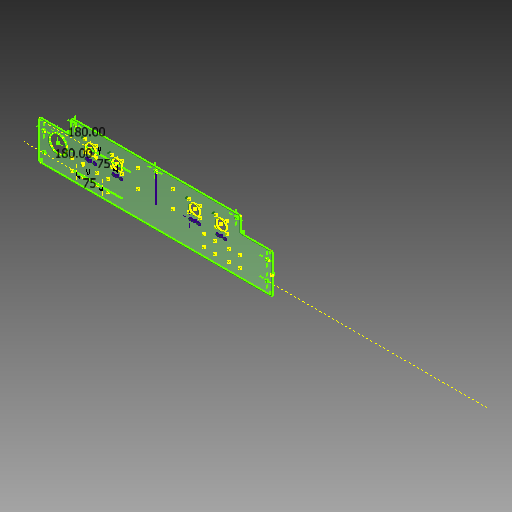
# Autodesk Inventor part: Rear Extruder Panel
Saved by Autodesk Inventor 2018 (Build 220112000, 112)
## iProperties
Created: 2016-06-26
Part Number: Rear Extruder Panel
Material: Polycarbonate, Smoke
Document SubType Name: Modeling
Designer: joshmamo
Density: 1.2 g/cm^3
Appearance: Polycarbonate - Clear(1)
Author: joshmamo
Autodesk Inventor part; units mm, degrees
ref_plane "YZ Plane" through (0, 0, 0) normal (1, 0, 0) x (0, 1, 0)
ref_plane "XZ Plane" through (0, 0, 0) normal (0, 1, 0) x (-1, 0, 0)
ref_plane "XY Plane" through (0, 0, 0) normal (0, 0, 1) x (1, 0, 0)
sketch "Sketch2" plane through (0, 0, 0) normal (0, 0, 1) x (1, 0, 0)
  line L0 (-94.6, 98.6888) -> (-564.8, 98.6888)
  line L1 (-89.6, 60.678) -> (-89.6, 93.6888)
  line L2 (-5, 55.678) -> (-84.6, 55.678)
  line L3 (0, -48.6888) -> (0, 48.6888)
  line L4 (-655, -53.6888) -> (-5, -53.6888)
  line L5 (-660, 50.6888) -> (-660, -48.6888)
  line L6 (-574.8, 55.6888) -> (-655, 55.6888)
  line L7 (-569.8, 93.6888) -> (-569.8, 60.6888)
  line L8 (-94.6, 98.6888) -> (-564.8, 98.6888)
  line L9 (-569.8, 93.6888) -> (-569.8, 60.6888)
  line L10 (-574.8, 55.6888) -> (-655, 55.6888)
  line L11 (-660, 50.6888) -> (-660, -48.6888)
  line L12 (-655, -53.6888) -> (-5, -53.6888)
  line L13 (0, -48.6888) -> (0, 50.678)
  line L14 (-5, 55.678) -> (-84.6, 55.678)
  line L15 (-89.6, 60.678) -> (-89.6, 93.6888)
  arc A0 (-89.6, 93.6888) -> (-94.6, 98.6888) centre (-94.6, 93.6888) ccw
  arc A1 (-89.6, 60.678) -> (-84.6, 55.678) centre (-84.6, 60.678) ccw
  arc A2 (0, 50.678) -> (-5, 55.678) centre (-5, 50.678) ccw
  arc A3 (-5, -53.6888) -> (0, -48.6888) centre (-5, -48.6888) ccw
  arc A4 (-660, -48.6888) -> (-655, -53.6888) centre (-655, -48.6888) ccw
  arc A5 (-655, 55.6888) -> (-660, 50.6888) centre (-655, 50.6888) ccw
  arc A6 (-574.8, 55.6888) -> (-569.8, 60.6888) centre (-574.8, 60.6888) ccw
  arc A7 (-564.8, 98.6888) -> (-569.8, 93.6888) centre (-564.8, 93.6888) ccw
  circle A8 centre (-605.9899, 16.8231) radius 24.5048
  line L16 (-17.508, -23.922) -> (609.984, -23.922) construction
  circle A9 centre (-645, 28.378) radius 2.55
  circle A10 centre (-645, -23.922) radius 2.55
  circle A11 centre (-557.8, 87.2888) radius 2.55
  circle A12 centre (-329.8, 87.2888) radius 2.55
  circle A13 centre (-101.8, 87.2888) radius 2.55
  circle A14 centre (-15, 28.378) radius 2.55
  circle A15 centre (-15, -23.922) radius 2.55
  point P0 (0, 0)
  point P1 (-581.4851, 16.8231)
  point P2 (-605.9899, 41.3279)
  point P3 (-560.308, 87.2888)
  point P4 (-557.8, 89.7968)
  point P5 (-645, 30.8968)
  point P6 (-647.508, 28.3888)
  point P7 (-329.8, 89.7968)
  point P8 (-332.308, 87.2888)
  point P9 (-101.8, 89.7968)
  point P10 (-104.308, 87.2888)
  point P11 (-15, 30.886)
  point P12 (-17.508, 28.378)
  point P13 (-15, -21.414)
  constraints: 37 end point, 16 point on circle, 15 centre point, 14 point on line, 1 horizontal, 1 vertical alignment, 2 other
sketch "Sketch3" plane through (0, 0, 0) normal (0, 0, 1) x (1, 0, 0)
  line L0 (-94.6, 98.6888) -> (-564.8, 98.6888)
  arc A0 (-564.8, 98.6888) -> (-569.8, 93.6888) centre (-564.8, 93.6888) ccw
  line L1 (-94.6, 98.6888) -> (-564.8, 98.6888)
  line L2 (-569.8, 93.6888) -> (-569.8, 60.6888)
  arc A1 (-574.8, 55.6888) -> (-569.8, 60.6888) centre (-574.8, 60.6888) ccw
  line L3 (-574.8, 55.6888) -> (-655, 55.6888)
  arc A2 (-655, 55.6888) -> (-660, 50.6888) centre (-655, 50.6888) ccw
  line L4 (-660, 50.6888) -> (-660, -48.6888)
  arc A3 (-660, -48.6888) -> (-655, -53.6888) centre (-655, -48.6888) ccw
  line L5 (-655, -53.6888) -> (-5, -53.6888)
  circle A4 centre (-605.9899, 16.8231) radius 24.5048
  circle A5 centre (-645, -23.922) radius 2.55
  circle A6 centre (-645, 28.378) radius 2.55
  circle A7 centre (-557.8, 87.2888) radius 2.55
  circle A8 centre (-329.8, 87.2888) radius 2.55
  circle A9 centre (-101.8, 87.2888) radius 2.55
  circle A10 centre (-15, 28.378) radius 2.55
  circle A11 centre (-15, -23.922) radius 2.55
  arc A12 (-5, -53.6888) -> (0, -48.6888) centre (-5, -48.6888) ccw
  line L6 (0, -48.6888) -> (0, 48.6888)
  arc A13 (0, 50.678) -> (-5, 55.678) centre (-5, 50.678) ccw
  line L7 (-5, 55.678) -> (-84.6, 55.678)
  arc A14 (-89.6, 60.678) -> (-84.6, 55.678) centre (-84.6, 60.678) ccw
  line L8 (-89.6, 60.678) -> (-89.6, 93.6888)
  arc A15 (-89.6, 93.6888) -> (-94.6, 98.6888) centre (-94.6, 93.6888) ccw
  point P0 (0, 0)
  constraints: 18 end point, 16 centre point, 16 point on circle
sketch "Sketch4" plane through (0, 0, 0) normal (0, 0, 1) x (1, 0, 0)
  line L0 (-94.6, 98.6888) -> (-564.8, 98.6888) projected
  arc A0 (-89.6, 93.6888) -> (-94.6, 98.6888) centre (-94.6, 93.6888) ccw projected
  line L1 (-89.6, 60.678) -> (-89.6, 93.6888) projected
  arc A1 (-89.6, 60.678) -> (-84.6, 55.678) centre (-84.6, 60.678) ccw projected
  line L2 (-5, 55.678) -> (-84.6, 55.678) projected
  arc A2 (0, 50.678) -> (-5, 55.678) centre (-5, 50.678) ccw projected
  line L3 (0, -48.6888) -> (0, 50.678) projected
  arc A3 (-5, -53.6888) -> (0, -48.6888) centre (-5, -48.6888) ccw projected
  line L4 (-655, -53.6888) -> (-5, -53.6888) projected
  arc A4 (-660, -48.6888) -> (-655, -53.6888) centre (-655, -48.6888) ccw projected
  line L5 (-660, 50.6888) -> (-660, -48.6888) projected
  arc A5 (-655, 55.6888) -> (-660, 50.6888) centre (-655, 50.6888) ccw projected
  line L6 (-574.8, 55.6888) -> (-655, 55.6888) projected
  arc A6 (-574.8, 55.6888) -> (-569.8, 60.6888) centre (-574.8, 60.6888) ccw projected
  line L7 (-569.8, 93.6888) -> (-569.8, 60.6888) projected
  arc A7 (-564.8, 98.6888) -> (-569.8, 93.6888) centre (-564.8, 93.6888) ccw projected
  point P0 (0, 0)
extrude "Extrusion1" add sketch "Sketch4" along normal blind 3
extrude "Extrusion2" cut sketch "Sketch3" along normal blind 3
sketch "Sketch5" plane through (0, 0, 0) normal (0, 0, -1) x (-1, 0, 0)
  line L0 (562.0823, -27.0183) -> (423.5029, -27.0183)
  line L1 (562.0823, -27.0183) -> (700.6617, -27.0183) construction
  line L2 (524.9252, 49.2029) -> (403.8589, 49.2029)
  line L3 (524.9252, 49.2029) -> (645.9914, 49.2029) construction
  line L4 (403.8589, 49.2029) -> (514.2755, 49.2029)
  line L5 (514.2755, 49.2029) -> (439.2755, 49.2029)
  line L6 (554.3408, -27.0183) -> (479.3408, -27.0183)
  point P0 (0, 0)
  dimension "d13" = 180
  dimension "d14" = 180
  dimension "d15" = 75
  dimension "d16" = 75
  constraints: 14 end point, 4 point on line, 2 collinear, 2 horizontal
  measures "d13" angle of L0 L1
  measures "d14" angle of L2 L3
  measures "d15" distance of L4.end L5.end
  measures "d16" distance of L6.start L6.end
sketch "Sketch6" plane through (0, 0, 0) normal (0, 0, -1) x (-1, 0, 0)
  circle A0 centre (529.7755, 64.7029) radius 1.7254
  circle A1 centre (498.7755, 64.7029) radius 1.6
  circle A2 centre (454.7755, 64.7029) radius 1.7254
  circle A3 centre (423.7755, 64.7029) radius 1.6
  spline S0 degree 3 number of poles 70
  circle A4 centre (498.7755, 33.6984) radius 1.6
  circle A5 centre (529.7755, 33.6984) radius 1.6
  circle A6 centre (529.7755, 64.7029) radius 1.6
  circle A7 centre (498.7755, 64.7029) radius 1.6
  circle A8 centre (454.7755, 33.6984) radius 1.6
  circle A9 centre (423.7755, 33.6984) radius 1.6
  circle A10 centre (454.7755, 64.7029) radius 1.6
  circle A11 centre (423.7755, 64.7029) radius 1.6
  circle A12 centre (329.8, 87.2888) radius 2.55
  line L0 (329.8, 87.2888) -> (329.8, 46.3988)
  point P0 (0, 0)
  point P1 (569.8408, -11.5183)
  point P2 (538.8408, -11.5183)
  point P3 (494.8408, -11.5183)
  point P4 (463.8408, -11.5183)
  point P5 (569.8408, -42.5229)
  point P6 (538.8408, -42.5229)
  point P7 (494.8408, -42.5229)
  point P8 (463.8408, -42.5229)
  point P9 (497.2709, 33.6984)
  point P10 (129.8245, 64.7029)
  point P11 (204.8245, 64.7029)
  point P12 (235.8245, 64.7029)
  point P13 (160.8245, 33.6984)
  point P14 (129.8245, 33.6984)
  point P15 (160.8245, 64.7029)
  point P16 (204.8245, 33.6984)
  point P17 (235.8245, 33.6984)
  dimension "d25" = 3.2
  dimension "d26" = 3.2
  dimension "d27" = 3.2
  dimension "d28" = 3.2
  dimension "d29" = 3.2
  dimension "d30" = 3.2
  dimension "d31" = 3.2
  dimension "d32" = 3.2
  constraints: 8 centre point, 8 symmetric about line, 4 coincident, 2 end point, 1 vertical
  measures "d25" diameter of A4
  measures "d26" diameter of A5
  measures "d27" diameter of A6
  measures "d28" diameter of A7
  measures "d29" diameter of A8
  measures "d30" diameter of A9
  measures "d31" diameter of A10
  measures "d32" diameter of A11
sketch "Sketch7" plane through (0, 0, 0) normal (0, 0, -1) x (-1, 0, 0)
  point P0 (0, 0)
  point P1 (554.3408, -27.0183)
  point P2 (479.3408, -27.0183)
  point P3 (439.2755, 49.2029)
  point P4 (514.2755, 49.2029)
sketch "Sketch8" plane through (0, 0, 0) normal (0, 0, -1) x (-1, 0, 0)
  circle A0 centre (439.2755, 49.2029) radius 14.5 projected
  circle A1 centre (514.2755, 49.2029) radius 14.5 projected
  circle A2 centre (329.8, 87.2888) radius 2.55 projected
  line L0 (329.8, 87.2888) -> (329.8, 25.8956)
  circle A3 centre (220.3245, 49.2029) radius 14.5
  circle A4 centre (145.3245, 49.2029) radius 14.5
  point P0 (0, 0)
  constraints: 2 end point, 2 symmetric about line, 1 vertical, 2 other
extrude "Extrusion3" cut sketch "Sketch8" against normal through all contours A0 | A1 | A3 | A4
sketch "Sketch9" plane through (0, 0, 0) normal (0, 0, -1) x (-1, 0, 0)
  circle A0 centre (329.8, 87.2888) radius 2.55 projected
  line L0 (329.8, 87.2888) -> (329.8, 5.9494)
  point P0 (0, 0)
  constraints: 2 end point, 1 vertical
hole "Hole2" at (-423.7755, 64.7029, 0) at (-423.7755, 33.6984, 0) at (-454.7755, 33.6984, 0) at (-454.7755, 64.7029, 0) at (-498.7755, 33.6984, 0) at (-498.7755, 64.7029, 0) at (-529.7755, 64.7029, 0) at (-529.7755, 33.6984, 0) at (-235.8245, 64.7029, 0) at (-204.8245, 64.7029, 0) at (-204.8245, 33.6984, 0) at (-235.8245, 33.6984, 0) at (-160.8245, 33.6984, 0) at (-160.8245, 64.7029, 0) at (-129.8245, 64.7029, 0) at (-129.8245, 33.6984, 0) direction (0, 0, 1) diameter 3 end through all
sketch "Sketch10" plane through (0, 0, 0) normal (0, 0, -1) x (-1, 0, 0)
  line L0 (329.8, 87.2888) -> (329.8, 5.9494) projected
  line L1 (329.8, 68.5151) -> (279.8, 68.5151)
  line L2 (329.8, 68.5151) -> (329.8, 18.5151)
  line L3 (329.8, 18.5151) -> (279.8, 18.5151)
  line L4 (279.8, 18.5151) -> (379.8, 18.5151)
  line L5 (379.8, 18.5151) -> (379.8, 68.5151)
  line L6 (329.8, 0) -> (91.883, 0)
  line L7 (91.883, 0) -> (91.883, -31.05)
  line L8 (91.883, -31.05) -> (122.933, -31.05)
  line L9 (91.883, 0) -> (122.933, 0)
  line L10 (122.933, 0) -> (162.933, 0)
  line L11 (162.933, 0) -> (162.933, -31.05)
  line L12 (162.933, -31.05) -> (193.983, -31.05)
  line L13 (567.717, 0) -> (567.717, -31.05)
  line L14 (567.717, -31.05) -> (536.667, -31.05)
  line L15 (496.667, 0) -> (496.667, -31.05)
  line L16 (496.667, -31.05) -> (465.617, -31.05)
  point P0 (0, 0)
  point P1 (193.983, 0)
  point P2 (536.667, 0)
  point P3 (465.617, 0)
  dimension "d49" = 50
  dimension "d50" = 50
  dimension "d51" = 100
  dimension "d52" = 31.05
  dimension "d53" = 31.05
  dimension "d54" = 40
  dimension "d55" = 31.05
  dimension "d56" = 31.05
  constraints: 32 end point, 8 symmetric about line, 5 point on line, 4 perpendicular, 3 horizontal
  measures "d49" distance of L1.start L1.end
  measures "d50" distance of L1.start L2.end
  measures "d51" distance of L3.end L4.end
  measures "d52" distance of L6.end L7.end
  measures "d53" distance of L7.end L8.end
  measures "d54" distance of L9.end L10.end
  measures "d55" distance of L11.start L11.end
  measures "d56" distance of L11.end L12.end
hole "Hole3" at (-91.883, 0, 0) at (-91.883, -31.05, 0) at (-122.933, -31.05, 0) at (-122.933, 0, 0) at (-162.933, 0, 0) at (-162.933, -31.05, 0) at (-193.983, -31.05, 0) at (-193.983, 0, 0) at (-279.8, 18.5151, 0) at (-279.8, 68.5151, 0) at (-379.8, 68.5151, 0) at (-379.8, 18.5151, 0) at (-496.667, 0, 0) at (-496.667, -31.05, 0) at (-465.617, -31.05, 0) at (-465.617, 0, 0) at (-536.667, 0, 0) at (-567.717, 0, 0) at (-567.717, -31.05, 0) at (-536.667, -31.05, 0) direction (0, 0, 1) diameter 3 end through all
sketch "Sketch11" plane through (0, 0, 0) normal (0, 0, -1) x (-1, 0, 0)
  circle A0 centre (567.717, -31.05) radius 1.5 projected
  circle A1 centre (536.667, 0) radius 1.5 projected
  circle A2 centre (465.617, -31.05) radius 1.5 projected
  circle A3 centre (496.667, 0) radius 1.5 projected
  circle A4 centre (379.8, 68.5151) radius 1.5 projected
  circle A5 centre (279.8, 18.5151) radius 1.5 projected
  circle A6 centre (193.983, -31.05) radius 1.5 projected
  circle A7 centre (162.933, 0) radius 1.5 projected
  circle A8 centre (122.933, -31.05) radius 1.5 projected
  circle A9 centre (91.883, 0) radius 1.5 projected
  circle A10 centre (91.883, -31.05) radius 1.5 projected
  circle A11 centre (122.933, 0) radius 1.5 projected
  circle A12 centre (162.933, -31.05) radius 1.5 projected
  circle A13 centre (193.983, 0) radius 1.5 projected
  circle A14 centre (279.8, 68.5151) radius 1.5 projected
  circle A15 centre (379.8, 18.5151) radius 1.5 projected
  circle A16 centre (496.667, -31.05) radius 1.5 projected
  circle A17 centre (465.617, 0) radius 1.5 projected
  circle A18 centre (567.717, 0) radius 1.5 projected
  circle A19 centre (536.667, -31.05) radius 1.5 projected
  circle A20 centre (129.8245, 64.7029) radius 1.5 projected
  circle A21 centre (160.8245, 33.6984) radius 1.5 projected
  circle A22 centre (204.8245, 33.6984) radius 1.5 projected
  circle A23 centre (235.8245, 64.7029) radius 1.5 projected
  circle A24 centre (529.7755, 64.7029) radius 1.5 projected
  circle A25 centre (498.7755, 33.6984) radius 1.5 projected
  circle A26 centre (454.7755, 33.6984) radius 1.5 projected
  circle A27 centre (423.7755, 64.7029) radius 1.5 projected
  circle A28 centre (423.7755, 33.6984) radius 1.5 projected
  circle A29 centre (454.7755, 64.7029) radius 1.5 projected
  circle A30 centre (498.7755, 64.7029) radius 1.5 projected
  circle A31 centre (529.7755, 33.6984) radius 1.5 projected
  circle A32 centre (204.8245, 64.7029) radius 1.5 projected
  circle A33 centre (235.8245, 33.6984) radius 1.5 projected
  circle A34 centre (160.8245, 64.7029) radius 1.5 projected
  circle A35 centre (129.8245, 33.6984) radius 1.5 projected
  circle A36 centre (220.3245, 49.2029) radius 14.5 projected
  circle A37 centre (439.2755, 49.2029) radius 14.5 projected
  circle A38 centre (514.2755, 49.2029) radius 14.5 projected
  circle A39 centre (145.3245, 49.2029) radius 14.5 projected
  circle A40 centre (15, -23.922) radius 2.55 projected
  circle A41 centre (101.8, 87.2888) radius 2.55 projected
  circle A42 centre (557.8, 87.2888) radius 2.55 projected
  circle A43 centre (645, -23.922) radius 2.55 projected
  circle A44 centre (645, 28.378) radius 2.55 projected
  circle A45 centre (329.8, 87.2888) radius 2.55 projected
  circle A46 centre (15, 28.378) radius 2.55 projected
  circle A47 centre (605.9899, 16.8231) radius 24.5048 projected
  line L0 (94.6, 98.6888) -> (564.8, 98.6888) projected
  arc A48 (94.6, 98.6888) -> (89.6, 93.6888) centre (94.6, 93.6888) ccw projected
  line L1 (89.6, 60.678) -> (89.6, 93.6888) projected
  arc A49 (84.6, 55.678) -> (89.6, 60.678) centre (84.6, 60.678) ccw projected
  line L2 (5, 55.678) -> (84.6, 55.678) projected
  arc A50 (5, 55.678) -> (0, 50.678) centre (5, 50.678) ccw projected
  line L3 (0, -48.6888) -> (0, 50.678) projected
  arc A51 (0, -48.6888) -> (5, -53.6888) centre (5, -48.6888) ccw projected
  line L4 (655, -53.6888) -> (5, -53.6888) projected
  arc A52 (655, -53.6888) -> (660, -48.6888) centre (655, -48.6888) ccw projected
  line L5 (660, 50.6888) -> (660, -48.6888) projected
  arc A53 (660, 50.6888) -> (655, 55.6888) centre (655, 50.6888) ccw projected
  line L6 (574.8, 55.6888) -> (655, 55.6888) projected
  arc A54 (569.8, 60.6888) -> (574.8, 55.6888) centre (574.8, 60.6888) ccw projected
  line L7 (569.8, 93.6888) -> (569.8, 60.6888) projected
  arc A55 (569.8, 93.6888) -> (564.8, 98.6888) centre (564.8, 93.6888) ccw projected
  circle A56 centre (145.3245, 19.7029) radius 1.6
  line L8 (137.8245, 17.6529) -> (131.6245, 17.6529)
  line L9 (137.8245, 21.7529) -> (137.8245, 17.6529)
  line L10 (131.6245, 21.7529) -> (137.8245, 21.7529)
  line L11 (131.6245, 17.6529) -> (131.6245, 21.7529)
  circle A57 centre (145.3245, 19.7029) radius 1.6
  line L12 (152.8245, 17.6529) -> (159.0245, 17.6529)
  line L13 (159.0245, 17.6529) -> (159.0245, 21.7529)
  line L14 (159.0245, 21.7529) -> (152.8245, 21.7529)
  line L15 (152.8245, 21.7529) -> (152.8245, 17.6529)
  line L16 (212.8245, 17.6529) -> (206.6245, 17.6529)
  line L17 (206.6245, 17.6529) -> (206.6245, 21.7529)
  line L18 (206.6245, 21.7529) -> (212.8245, 21.7529)
  line L19 (212.8245, 21.7529) -> (212.8245, 17.6529)
  circle A58 centre (220.3245, 19.7029) radius 1.6
  line L20 (227.8245, 17.6529) -> (234.0245, 17.6529)
  line L21 (234.0245, 17.6529) -> (234.0245, 21.7529)
  line L22 (234.0245, 21.7529) -> (227.8245, 21.7529)
  line L23 (227.8245, 21.7529) -> (227.8245, 17.6529)
  circle A59 centre (439.2755, 19.7029) radius 1.6
  line L24 (431.7755, 21.7529) -> (431.7755, 17.6529)
  line L25 (431.7755, 17.6529) -> (425.5755, 17.6529)
  line L26 (425.5755, 17.6529) -> (425.5755, 21.7529)
  line L27 (425.5755, 21.7529) -> (431.7755, 21.7529)
  line L28 (446.7755, 21.7529) -> (446.7755, 17.6529)
  line L29 (446.7755, 17.6529) -> (452.9755, 17.6529)
  line L30 (452.9755, 17.6529) -> (452.9755, 21.7529)
  line L31 (452.9755, 21.7529) -> (446.7755, 21.7529)
  line L32 (506.7755, 17.6529) -> (500.5755, 17.6529)
  line L33 (506.7755, 21.7529) -> (506.7755, 17.6529)
  line L34 (500.5755, 21.7529) -> (506.7755, 21.7529)
  line L35 (500.5755, 17.6529) -> (500.5755, 21.7529)
  circle A60 centre (514.2755, 19.7029) radius 1.6
  line L36 (521.7755, 17.6529) -> (527.9755, 17.6529)
  line L37 (527.9755, 17.6529) -> (527.9755, 21.7529)
  line L38 (527.9755, 21.7529) -> (521.7755, 21.7529)
  line L39 (521.7755, 21.7529) -> (521.7755, 17.6529)
  point P0 (0, 0)
  constraints: 64 end point, 16 horizontal, 16 vertical, 5 centre point, 43 other
sketch "Sketch13" plane through (0, 0, 0) normal (0, 0, -1) x (-1, 0, 0)
  circle A0 centre (145.3245, 19.7029) radius 1.6 projected
  line L0 (152.9245, 21.2029) -> (158.9245, 21.2029) projected
  line L1 (158.9245, 21.2029) -> (158.9245, 18.2029) projected
  line L2 (152.9245, 18.2029) -> (152.9245, 21.2029) projected
  line L3 (158.9245, 18.2029) -> (152.9245, 18.2029) projected
  line L4 (137.7245, 21.2029) -> (137.7245, 18.2029) projected
  line L5 (131.7245, 21.2029) -> (137.7245, 21.2029) projected
  line L6 (131.7245, 18.2029) -> (131.7245, 21.2029) projected
  line L7 (137.7245, 18.2029) -> (131.7245, 18.2029) projected
  point P0 (0, 0)
extrude "Extrusion5" cut sketch "Sketch13" against normal through all
pattern_linear "Rectangular Pattern1" count 2 spacing 75 along (-1, 0, 0) of "Extrusion5"
pattern_linear "Rectangular Pattern2" count 2 spacing 294 along (-1, 0, 0) of "Extrusion5"
pattern_linear "Rectangular Pattern3" count 2 spacing 75 along (-1, 0, 0) of "Rectangular Pattern2"
sketch "Sketch14" plane through (0, 0, 3) normal (0, 0, 1) x (1, 0, 0)
  point P0 (0, 0)
sketch "Sketch15" plane through (0, 0, 3) normal (0, 0, 1) x (1, 0, 0)
  arc A0 (-462.0622, 65.7187) -> (-461.1816, 65.3945) centre (-461.5622, 65.7187) ccw projected
  line L0 (-461.1816, 65.3945) -> (-460.3625, 66.3563) projected
  line L1 (-460.3625, 66.3563) -> (-457.3793, 69.2691) projected
  arc A1 (-457.3793, 69.2691) -> (-457.7286, 70.1268) centre (-457.7286, 69.6268) ccw projected
  line L2 (-457.7286, 70.1268) -> (-459.0622, 70.1268) projected
  arc A2 (-459.0622, 70.1268) -> (-462.0622, 67.1268) centre (-459.0622, 67.1268) ccw projected
  line L3 (-462.0622, 67.1268) -> (-462.0622, 65.7187) projected
  arc A3 (-534.0622, 70.1268) -> (-537.0622, 67.1268) centre (-534.0622, 67.1268) ccw projected
  line L4 (-537.0622, 67.1268) -> (-537.0622, 65.7187) projected
  arc A4 (-537.0622, 65.7187) -> (-536.1816, 65.3945) centre (-536.5622, 65.7187) ccw projected
  line L5 (-536.1816, 65.3945) -> (-535.3625, 66.3563) projected
  line L6 (-535.3625, 66.3563) -> (-532.3793, 69.2691) projected
  arc A5 (-532.3793, 69.2691) -> (-532.7286, 70.1268) centre (-532.7286, 69.6268) ccw projected
  line L7 (-532.7286, 70.1268) -> (-534.0622, 70.1268) projected
  circle A6 centre (-454.7755, 64.7029) radius 1.5 projected
  point P0 (0, 0)
  constraints: 1 coincident
extrude "Extrusion6" cut sketch "Sketch15" against normal blind 10 contours L3 A2 L2 A1 L1 L0 A0 | L7 A5 L6 L5 A4 L4 A3
sketch "Sketch16" plane through (0, 0, 3) normal (0, 0, 1) x (1, 0, 0)
  arc A0 (-459.0622, 70.1268) -> (-462.0622, 67.1268) centre (-459.0622, 67.1268) ccw projected
  line L0 (-462.0622, 67.1268) -> (-462.0622, 65.7187) projected
  arc A1 (-462.0622, 65.7187) -> (-461.1816, 65.3945) centre (-461.5622, 65.7187) ccw projected
  line L1 (-461.1816, 65.3945) -> (-460.3625, 66.3563) projected
  line L2 (-460.3625, 66.3563) -> (-457.3793, 69.2691) projected
  arc A2 (-457.3793, 69.2691) -> (-457.7286, 70.1268) centre (-457.7286, 69.6268) ccw projected
  line L3 (-457.7286, 70.1268) -> (-459.0622, 70.1268) projected
  line L4 (-459.0622, 70.1268) -> (-457.7286, 70.1268) projected
  line L5 (-459.0622, 70.1268) -> (-457.7286, 70.1268)
  line L6 (-460.3625, 66.3563) -> (-457.3793, 69.2691) projected
  line L7 (-457.3793, 69.2691) -> (-460.3625, 66.3563)
  line L8 (-460.3625, 66.3563) -> (-461.1816, 65.3945) projected
  line L9 (-460.3625, 66.3563) -> (-461.1816, 65.3945)
  line L10 (-462.0622, 65.7187) -> (-462.0622, 67.1268) projected
  line L11 (-462.0622, 65.7187) -> (-462.0622, 67.1268)
  arc A3 (-459.0622, 70.1268) -> (-462.0622, 67.1268) centre (-459.0622, 67.1268) ccw projected
  arc A4 (-459.0622, 70.1268) -> (-462.0622, 67.1268) centre (-459.0622, 67.1268) ccw
  arc A5 (-457.3793, 69.2691) -> (-457.7286, 70.1268) centre (-457.7286, 69.6268) ccw projected
  arc A6 (-459.0622, 70.1268) -> (-462.0622, 67.1268) centre (-459.0622, 67.1268) ccw
  arc A7 (-457.3793, 69.2691) -> (-457.7286, 70.1268) centre (-457.7286, 69.6268) ccw
  arc A8 (-462.0622, 65.7187) -> (-461.1816, 65.3945) centre (-461.5622, 65.7187) ccw
  line L12 (-240.1097, 70.1268) -> (-238.7761, 70.1268)
  line L13 (-238.4268, 69.2691) -> (-241.41, 66.3563)
  line L14 (-241.41, 66.3563) -> (-242.2291, 65.3945)
  line L15 (-243.1097, 65.7187) -> (-243.1097, 67.1268)
  arc A9 (-240.1097, 70.1268) -> (-243.1097, 67.1268) centre (-240.1097, 67.1268) ccw
  arc A10 (-240.1097, 70.1268) -> (-243.1097, 67.1268) centre (-240.1097, 67.1268) ccw
  arc A11 (-238.4268, 69.2691) -> (-238.7761, 70.1268) centre (-238.7761, 69.6268) ccw
  arc A12 (-243.1097, 65.7187) -> (-242.2291, 65.3945) centre (-242.6097, 65.7187) ccw
  line L16 (-165.1194, 70.1268) -> (-163.7858, 70.1268)
  line L17 (-163.4365, 69.2691) -> (-166.4196, 66.3563)
  line L18 (-166.4196, 66.3563) -> (-167.2387, 65.3945)
  line L19 (-168.1194, 65.7187) -> (-168.1194, 67.1268)
  arc A13 (-165.1194, 70.1268) -> (-168.1194, 67.1268) centre (-165.1194, 67.1268) ccw
  arc A14 (-165.1194, 70.1268) -> (-168.1194, 67.1268) centre (-165.1194, 67.1268) ccw
  arc A15 (-163.4365, 69.2691) -> (-163.7858, 70.1268) centre (-163.7858, 69.6268) ccw
  arc A16 (-168.1194, 65.7187) -> (-167.2387, 65.3945) centre (-167.6194, 65.7187) ccw
  point P0 (0, 0)
  point P1 (-454.7755, 64.7029)
  point P2 (-454.7755, 64.7029)
  point P3 (-235.823, 64.7029)
  point P4 (-160.8326, 64.7029)
  constraints: 25 point on circle, 24 end point, 12 centre point, 6 point on line, 5 coincident, 4 collinear
extrude "Extrusion7" cut sketch "Sketch16" against normal blind 10 contours L12 A11 L13 L14 A12 L15 A9 | L16 A15 L17 L18 A16 L19 A13
sketch "Sketch17" plane through (0, 0, 3) normal (0, 0, 1) x (1, 0, 0)
  point P0 (0, 0)
body "Solid1"
